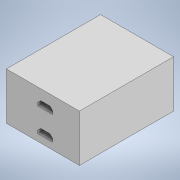
# Autodesk Inventor part: Contactile Communication Hub
Saved by Autodesk Inventor 2022 (Build 260153000, 153)
## iProperties
Created: 2021-09-20
Part Number: Contactile Communication Hub
Material: Generic
Document SubType Name: Modeling
Designer: kylem
Density: 1 g/cm^3
Appearance: Default
Author: kylem
Autodesk Inventor part; units mm, degrees
ref_plane "YZ Plane" through (0, 0, 0) normal (1, 0, 0) x (0, 1, 0)
ref_plane "XZ Plane" through (0, 0, 0) normal (0, 1, 0) x (-1, 0, 0)
ref_plane "XY Plane" through (0, 0, 0) normal (0, 0, 1) x (1, 0, 0)
sketch "Sketch1" plane through (0, 0, 0) normal (0, 1, 0) x (-1, 0, 0)
  line L0 (0, 0) -> (38, 0)
  line L1 (38, 0) -> (38, -49)
  line L2 (38, -49) -> (0, -49)
  line L3 (0, -49) -> (0, 0)
  dimension "d0" = 38
  dimension "d1" = 49
  constraints: 8 end point, 2 parallel, 1 horizontal, 1 perpendicular
  measures "d0" distance of L1.end L2.end
  measures "d1" distance of L0.end L1.end
extrude "Extrusion1" add sketch "Sketch1" along normal blind 24.5
sketch "Sketch3" plane through (-38, 0, -49) normal (-1, 0, 0) x (0, 0, 1)
  line L0 (0, 0) -> (0, 24.5) projected
  line L1 (0, 0) -> (0, 15.1)
  line L2 (0, 15.1) -> (6.1, 15.1)
  line L3 (6.1, 15.1) -> (23.1, 15.1)
  line L4 (23.1, 15.1) -> (23.1, 19)
  line L5 (23.1, 19) -> (6.1, 19)
  line L6 (6.1, 19) -> (6.1, 15.1)
  line L7 (0, 0) -> (49, 0) projected
  line L8 (0, 0) -> (49, 0)
  line L9 (24.5, 0) -> (24.5, -2.7502)
  line L10 (49, 15.1) -> (42.9, 15.1)
  line L11 (42.9, 15.1) -> (25.9, 15.1)
  line L12 (25.9, 15.1) -> (25.9, 19)
  line L13 (25.9, 19) -> (42.9, 19)
  line L14 (42.9, 19) -> (42.9, 15.1)
  dimension "d8" = 15.1
  dimension "d9" = 6.1
  dimension "d10" = 17
  dimension "d11" = 3.9
  constraints: 26 end point, 5 symmetric about line, 2 horizontal, 2 parallel, 2 perpendicular, 1 midpoint, 1 point on line, 1 vertical
  measures "d8" distance of L0.start L1.end
  measures "d9" distance of L1.end L2.end
  measures "d10" distance of L5.end L4.end
  measures "d11" distance of L4.end L3.end
extrude "Extrusion2" cut sketch "Sketch3" against normal blind 15
sketch "Sketch4" plane through (-38, 0, 0) normal (0, 0, 1) x (1, 0, 0)
  line L0 (0, 0) -> (0, 24.5) projected
  line L1 (0, 24.5) -> (16.4, 24.5)
  line L2 (0, 24.5) -> (38, 24.5) projected
  line L3 (16.4, 24.5) -> (16.4, 16.15)
  line L4 (16.4, 16.15) -> (24.15, 16.15)
  line L5 (24.15, 16.15) -> (24.15, 19.15)
  line L6 (24.15, 19.15) -> (16.4, 19.15)
  line L7 (16.4, 19.15) -> (16.4, 16.15)
  line L8 (16.4, 16.15) -> (16.4, 3.65)
  line L9 (16.4, 3.65) -> (24.15, 3.65)
  line L10 (24.15, 3.65) -> (24.15, 6.65)
  line L11 (24.15, 6.65) -> (16.4, 6.65)
  line L12 (16.4, 6.65) -> (16.4, 3.65)
  point P0 (38, 0)
  point P1 (16.4, 6.65)
  point P2 (16.4, 19.15)
  dimension "d14" = 16.4
  dimension "d15" = 8.35
  dimension "d16" = 7.75
  dimension "d17" = 3
  dimension "d18" = 12.5
  dimension "d19" = 7.75
  dimension "d20" = 3
  constraints: 22 end point, 4 parallel, 2 horizontal, 2 perpendicular, 2 vertical, 1 point on line
  measures "d14" distance of L0.end L1.end
  measures "d15" distance of L1.end L3.end
  measures "d16" distance of L6.end L5.end
  measures "d17" distance of L5.end L4.end
  measures "d18" distance of L3.end L8.end
  measures "d19" distance of L11.end L10.end
  measures "d20" distance of L10.end L9.end
extrude "Extrusion3" cut sketch "Sketch4" against normal blind 15
chamfer "Chamfer1" distance 1.5 angle 45 4 edges at (-13.85, 19.15, -7.5) (-13.85, 6.65, -7.5) (-21.6, 19.15, -7.5) (-21.6, 6.65, -7.5)
sketch "Sketch5" plane through (0, 0, 0) normal (0, -1, 0) x (1, 0, 0)
  line L0 (-38, 0) -> (0, 0) projected
  line L1 (0, 0) -> (-4.75, 0)
  line L2 (-4.75, 0) -> (-4.75, -8.5)
  line L3 (-4.75, -8.5) -> (-4.75, -40.5)
  line L4 (-4.75, -40.5) -> (-33.25, -40.5)
  line L5 (-33.25, -40.5) -> (-33.25, -8.5)
  line L6 (-38, -6.1) -> (-23, -6.1) projected
  circle A0 centre (-33.25, -40.5) radius 1.5
  circle A1 centre (-4.75, -40.5) radius 1.5
  circle A2 centre (-4.75, -8.5) radius 1.5
  circle A3 centre (-33.25, -8.5) radius 1.5
  dimension "d26" = 4.75
  dimension "d27" = 8.5
  dimension "d28" = 32
  dimension "d29" = 28.5
  dimension "d30" = 3
  dimension "d31" = 3
  dimension "d32" = 3
  dimension "d33" = 3
  constraints: 10 end point, 4 centre point, 4 coincident, 3 perpendicular, 2 point on line
  measures "d26" distance of L0.end L1.end
  measures "d27" distance of L1.end L2.end
  measures "d28" distance of L2.end L3.end
  measures "d29" distance of L3.end L4.end
  measures "d30" diameter of A0
  measures "d31" diameter of A1
  measures "d32" diameter of A2
  measures "d33" diameter of A3
extrude "Extrusion4" cut sketch "Sketch5" against normal blind 10
body "Solid1"
